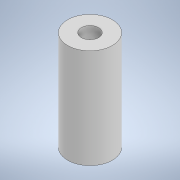
# Autodesk Inventor part: sepmoit
Saved by Autodesk Inventor 2022 (Build 260153000, 153)
## iProperties
Created: 2022-03-10
Part Number: sepmoit
Material: Genérico
Document SubType Name: Modeling
Designer: JK
Density: 1 g/cm^3
Appearance: Valor por defecto
Author: JK
Autodesk Inventor part; units mm, degrees
ref_plane "YZ Plane" through (0, 0, 0) normal (1, 0, 0) x (0, 1, 0)
ref_plane "XZ Plane" through (0, 0, 0) normal (0, 1, 0) x (-1, 0, 0)
ref_plane "XY Plane" through (0, 0, 0) normal (0, 0, 1) x (1, 0, 0)
sketch "Boceto1" plane through (0, 0, 0) normal (0, 1, 0) x (-1, 0, 0)
  circle A0 centre (0, 0) radius 4.5
  circle A1 centre (0, 0) radius 1.75
  dimension "d0" = 9
  dimension "d1" = 3.5
  constraints: 2 centre point, 2 coincident
  measures "d0" diameter of A0
  measures "d1" diameter of A1
extrude "Extrusión1" add sketch "Boceto1" along normal blind 20
